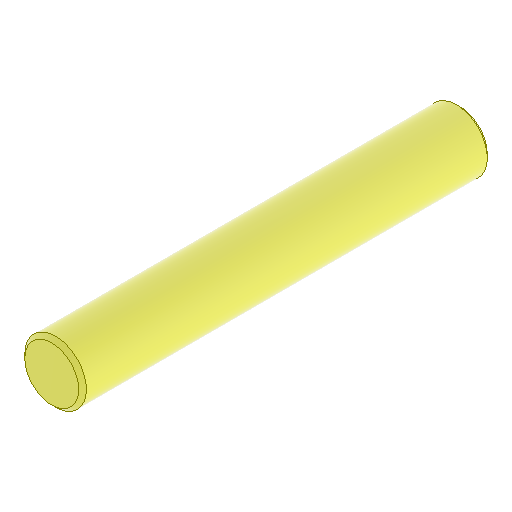
# Autodesk Inventor part: GRJ-05-104
Saved by Autodesk Inventor 2026.1 (Build 301233000, 233)
## iProperties
Company: Gree
Created: 2025-08-14
Part Number: GRJ-05-104
Material: Poliacetal WT
Document SubType Name: Modeling
Designer: Willian Pinheiro
Density: 1.4 g/cm^3
Appearance: Suave - Amarelo
Project: GRJ-05
Description: Coluna Apoio B
Mass: 3.61938 g
Surface Area: 15.3262 cm^2
Volume: 2.58527 cm^3
Checked By: Antonio Lucas
Engr Approved By: Antonio Lucas
Mfg Approved By: Anderson Oliveira
Acabamento: N/A
Dimensões: Ø8 x 53 mm
Total: 2
Author: Willian Pinheiro
Revision Number: 00
Title: Parafusamento
Autodesk Inventor part; units mm, degrees
ref_plane "YZ Plane" through (0, 0, 0) normal (1, 0, 0) x (0, 1, 0)
ref_plane "XZ Plane" through (0, 0, 0) normal (0, 1, 0) x (-1, 0, 0)
ref_plane "XY Plane" through (0, 0, 0) normal (0, 0, 1) x (1, 0, 0)
sketch "Sketch1" plane through (0, 0, 0) normal (0, 0, 1) x (1, 0, 0)
  line L0 (-4.8, 0) -> (0.8, 0) construction
  line L1 (0, -37.1) -> (0, 37.1) construction
  line L2 (-4, 26.5) -> (0, 26.5)
  line L3 (0, 26.5) -> (0, -26.5)
  line L4 (0, -26.5) -> (-4, -26.5)
  line L5 (-4, -26.5) -> (-4, 26.5)
  point P0 (0, 0)
  dimension "d1" = 53
  dimension "d16" = 8
  constraints: 8 end point, 2 parallel, 1 collinear, 1 horizontal, 1 perpendicular, 1 other
  measures "d1" distance between parallel lines of L4 L2
  measures "d16" diameter of L5 L1
revolve "Revolution1" add sketch "Sketch1" angle 360 about axis through (0, -10, 0) along (0, 1, 0)
sketch "Sketch2" plane through (0, 26.5, 0) normal (0, 1, 0) x (1, 0, 0)
  circle A0 centre (0, 0) radius 4 projected
  constraints: 1 coincident
hole "Hole1" at (0, 26.5, 0) direction (0, -1, 0) diameter 2.459 depth 15 tip angle 118 thread size "M3x0.5" class "6H" standard "ISO Metric profile"
mirror "Espelhar1" [suppressed]
chamfer "Chamfer1" distance 0.5 angle 45 2 edges at (4, -26.5, 0) (4, 26.5, 0)
chamfer "Chamfer2" distance 0.3 angle 45 1 edges at (0, 26.5, -1.2295)
body "Solid1"
